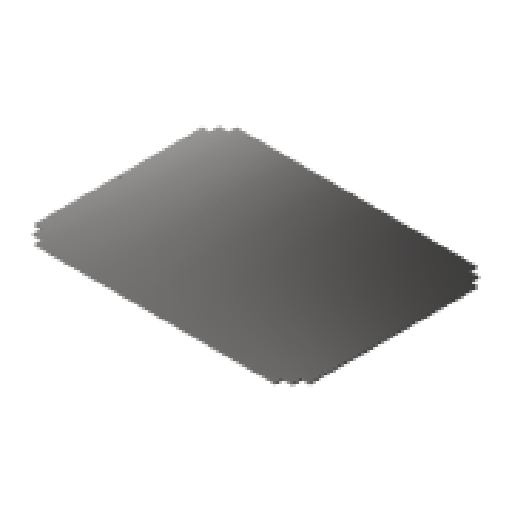
# Autodesk Inventor part: BasePlate
Saved by Autodesk Inventor 2023.2 (Build 272271000, 271)
## iProperties
Created: 2020-05-08
Part Number: BasePlate
Material: Aluminum 6061
Document SubType Name: Modeling
Designer: Remo
Mass: 4435.74 g
Surface Area: 3861.35 cm^2
Volume: 565.063 cm^3
Density: 2.7 g/cm^3
Appearance: Aluminum - Dark
Description: LaserTeileOnline / 3mm Aluminum / Base Plate
Author: Remo
Revision Number: 1
Autodesk Inventor part; units mm, degrees
ref_plane "YZ Plane" through (0, 0, 0) normal (1, 0, 0) x (0, 1, 0)
ref_plane "XZ Plane" through (0, 0, 0) normal (0, 1, 0) x (-1, 0, 0)
ref_plane "XY Plane" through (0, 0, 0) normal (0, 0, 1) x (1, 0, 0)
sketch "Sketch1" plane through (0, 0, 0) normal (0, 0, 1) x (1, 0, 0)
  line L0 (-412.8165, 301.8597) -> (87.1835, 301.8597) projected
  line L1 (-427.8165, 301.8597) -> (-412.8165, 301.8597) projected
  line L2 (-427.8165, 286.8597) -> (-427.8165, 301.8597) projected
  line L3 (-427.8165, -73.1403) -> (-427.8165, 286.8597) projected
  line L4 (-412.8165, 286.8597) -> (-427.8165, 286.8597) projected
  line L5 (-412.8165, 286.8597) -> (-427.8165, 286.8597) projected
  line L6 (-412.8165, 301.8597) -> (-412.8165, 286.8597) projected
  line L7 (-427.8165, 301.8597) -> (-412.8165, 301.8597) projected
  line L8 (-427.8165, 286.8597) -> (-427.8165, 301.8597) projected
  line L9 (-412.8165, -88.1403) -> (-412.8165, -73.1403) projected
  line L10 (-412.8165, -73.1403) -> (-427.8165, -73.1403) projected
  line L11 (-427.8165, -88.1403) -> (-427.8165, -73.1403) projected
  line L12 (-412.8165, -88.1403) -> (-427.8165, -88.1403) projected
  line L13 (-412.8165, -73.1403) -> (-412.8165, 286.8597) projected
  line L14 (87.1835, -73.1403) -> (-412.8165, -73.1403) projected
  line L15 (87.1835, -88.1403) -> (-412.8165, -88.1403) projected
  line L16 (102.1835, -88.1403) -> (102.1835, -73.1403) projected
  line L17 (102.1835, -73.1403) -> (87.1835, -73.1403) projected
  line L18 (87.1835, -88.1403) -> (87.1835, -73.1403) projected
  line L19 (102.1835, -88.1403) -> (87.1835, -88.1403) projected
  line L20 (87.1835, -73.1403) -> (87.1835, 286.8597) projected
  line L21 (102.1835, -73.1403) -> (102.1835, 286.8597) projected
  line L22 (87.1835, 286.8597) -> (102.1835, 286.8597) projected
  line L23 (102.1835, 286.8597) -> (102.1835, 301.8597) projected
  line L24 (87.1835, 301.8597) -> (102.1835, 301.8597) projected
  line L25 (87.1835, 286.8597) -> (87.1835, 301.8597) projected
  line L26 (87.1835, 286.8597) -> (-412.8165, 286.8597) projected
  line L27 (-312.8165, -73.1403) -> (-312.8165, 286.8597) projected
  line L28 (-297.8165, -73.1403) -> (-297.8165, 286.8597) projected
  line L29 (-12.8165, -73.1403) -> (-12.8165, 286.8597) projected
  line L30 (-27.8165, -73.1403) -> (-27.8165, 286.8597) projected
  line L31 (-425.8165, -71.1403) -> (-410.8165, -71.1403)
  line L32 (-410.8165, -71.1403) -> (-410.8165, -86.1403)
  line L33 (-410.8165, -86.1403) -> (85.1835, -86.1403)
  line L34 (85.1835, -86.1403) -> (85.1835, -71.1403)
  line L35 (85.1835, -71.1403) -> (100.1835, -71.1403)
  line L36 (100.1835, -71.1403) -> (100.1835, 284.8597)
  line L37 (100.1835, 284.8597) -> (85.1835, 284.8597)
  line L38 (85.1835, 284.8597) -> (85.1835, 299.8597)
  line L39 (85.1835, 299.8597) -> (-410.8165, 299.8597)
  line L40 (-410.8165, 299.8597) -> (-410.8165, 284.8597)
  line L41 (-410.8165, 284.8597) -> (-425.8165, 284.8597)
  line L42 (-425.8165, 284.8597) -> (-425.8165, -71.1403)
  point P0 (0, 0)
  dimension "d2" = 2
  dimension "d3" = 2
  dimension "d4" = 2
  dimension "d5" = 2
  dimension "d6" = 2
  dimension "d7" = 2
  dimension "d8" = 2
  dimension "d9" = 2
  dimension "d10" = 2
  dimension "d11" = 2
  dimension "d12" = 2
  dimension "d13" = 2
  constraints: 24 end point, 7 perpendicular, 4 parallel, 1 horizontal
  measures "d2" distance between parallel lines of L10 L31
  measures "d3" distance between parallel lines of L3 L42
  measures "d4" distance between parallel lines of L9 L32
  measures "d5" distance between parallel lines of L15 L33
  measures "d6" distance between parallel lines of L34 L18
  measures "d7" distance between parallel lines of L17 L35
  measures "d8" distance between parallel lines of L21 L36
  measures "d9" distance between parallel lines of L22 L37
  measures "d10" distance between parallel lines of L25 L38
  measures "d11" distance between parallel lines of L0 L39
  measures "d12" distance between parallel lines of L6 L40
  measures "d13" distance between parallel lines of L4 L41
extrude "Extrusion1" add sketch "Sketch1" along normal blind 3 contours L41 L40 L26 L27 L14 L32 L31 L13 | L13 L31 L42 L41 | L40 L39 L38 L26 | L37 L36 L35 L20 | L20 L35 L34 L14 L29 L26 L38 L37 | L26 L28 L14 L27 | L29 L14 L30 L26 | L26 L30 L14 L28 | L14 L34 L33 L32
sketch "Sketch3" plane through (0, 0, 3) normal (0, 0, 1) x (1, 0, 0)
  line L0 (100.1835, -71.1403) -> (100.1835, 284.8597) projected
  line L1 (-425.8165, 284.8597) -> (-425.8165, -71.1403) projected
  line L2 (-425.8165, -71.1403) -> (-410.8165, -71.1403) projected
  line L3 (-410.8165, 284.8597) -> (-425.8165, 284.8597) projected
  line L4 (85.1835, -86.1403) -> (85.1835, -71.1403) projected
  line L5 (-410.8165, 299.8597) -> (-410.8165, 284.8597) projected
  line L6 (-410.8165, -86.1403) -> (85.1835, -86.1403) projected
  line L7 (85.1835, 299.8597) -> (-410.8165, 299.8597) projected
  point P0 (0, 0)
  point P1 (94.6835, -21.1403)
  point P2 (94.6835, 106.8597)
  point P3 (94.6835, 234.8597)
  point P4 (-420.3165, 234.8597)
  point P5 (-420.3165, 106.8597)
  point P6 (-420.3165, -21.1403)
  point P7 (35.1835, -80.6403)
  point P8 (-94.8165, -80.6403)
  point P9 (-230.8165, -80.6403)
  point P10 (-360.8165, -80.6403)
  point P11 (-360.8165, 294.3597)
  point P12 (-230.8165, 294.3597)
  point P13 (-94.8165, 294.3597)
  point P14 (35.1835, 294.3597)
  dimension "d18" = 5.5
  dimension "d19" = 5.5
  dimension "d20" = 50
  dimension "d21" = 50
  dimension "d22" = 356
  dimension "d23" = 178
  dimension "d24" = 50
  dimension "d25" = 50
  dimension "d26" = 5.5
  dimension "d27" = 5.5
  dimension "d28" = 180
  dimension "d29" = 180
  constraints: 9 horizontal alignment, 8 vertical alignment
  measures "d18" distance from line of L0 point (94.684, -21.14)
  measures "d19" distance from line of L1 point (-420.316, -21.14)
  measures "d20" distance from line of L2 point (-420.316, -21.14)
  measures "d21" distance from line of L3 point (-420.316, 234.86)
  measures "d22" distance of L1.start L1.end
  measures "d23" distance from line of L2 point (-420.316, 106.86)
  measures "d24" distance from line of L4 point (35.184, -80.64)
  measures "d25" distance from line of L5 point (-360.816, 294.36)
  measures "d26" distance from line of L6 point (35.184, -80.64)
  measures "d27" distance from line of L7 point (35.184, 294.36)
  measures "d28" horizontal distance of L6.start point (-230.816, -80.64)
  measures "d29" distance from line of L4 point (-94.816, -80.64)
hole "FrameMountHoles" at (94.6835, -21.1403, 3) at (94.6835, 106.8597, 3) at (94.6835, 234.8597, 3) at (-420.3165, 234.8597, 3) at (-420.3165, 106.8597, 3) at (-420.3165, -21.1403, 3) at (35.1835, -80.6403, 3) at (-94.8165, -80.6403, 3) at (-230.8165, -80.6403, 3) at (-360.8165, -80.6403, 3) at (-360.8165, 294.3597, 3) at (-230.8165, 294.3597, 3) at (-94.8165, 294.3597, 3) at (35.1835, 294.3597, 3) direction (0, 0, -1) diameter 4 depth 8 tip angle 118
sketch "Sketch10" plane through (0, 0, 3) normal (0, 0, 1) x (1, 0, 0)
  circle A0 centre (-94.8165, 294.3597) radius 2 projected
  circle A1 centre (-360.8165, 294.3597) radius 2 projected
  circle A2 centre (-230.8165, -80.6403) radius 2 projected
  circle A3 centre (35.1835, -80.6403) radius 2 projected
  circle A4 centre (-420.3165, 106.8597) radius 2 projected
  circle A5 centre (94.6835, 234.8597) radius 2 projected
  circle A6 centre (94.6835, -21.1403) radius 2 projected
  circle A7 centre (94.6835, 106.8597) radius 2 projected
  circle A8 centre (-420.3165, 234.8597) radius 2 projected
  circle A9 centre (-420.3165, -21.1403) radius 2 projected
  circle A10 centre (-94.8165, -80.6403) radius 2 projected
  circle A11 centre (-360.8165, -80.6403) radius 2 projected
  circle A12 centre (-230.8165, 294.3597) radius 2 projected
  circle A13 centre (35.1835, 294.3597) radius 2 projected
  line L0 (-425.8165, -71.1403) -> (-410.8165, -71.1403) projected
  line L1 (-410.8165, -71.1403) -> (-410.8165, -86.1403) projected
  line L2 (-410.8165, -86.1403) -> (85.1835, -86.1403) projected
  line L3 (85.1835, -86.1403) -> (85.1835, -71.1403) projected
  line L4 (85.1835, -71.1403) -> (100.1835, -71.1403) projected
  line L5 (100.1835, -71.1403) -> (100.1835, 284.8597) projected
  line L6 (100.1835, 284.8597) -> (85.1835, 284.8597) projected
  line L7 (85.1835, 284.8597) -> (85.1835, 299.8597) projected
  line L8 (85.1835, 299.8597) -> (-410.8165, 299.8597) projected
  line L9 (-410.8165, 299.8597) -> (-410.8165, 284.8597) projected
  line L10 (-410.8165, 284.8597) -> (-425.8165, 284.8597) projected
  line L11 (-425.8165, 284.8597) -> (-425.8165, -71.1403) projected
  line L12 (100.1835, -71.1403) -> (100.1835, 284.8597) projected
  line L13 (85.1835, 284.8597) -> (100.1835, 284.8597)
  line L14 (100.1835, 284.8597) -> (100.1835, 266.8597)
  line L15 (100.1835, 266.8597) -> (85.1835, 266.8597)
  line L16 (85.1835, 266.8597) -> (85.1835, 284.8597)
  line L17 (85.1835, 284.8597) -> (67.1835, 284.8597)
  line L18 (67.1835, 284.8597) -> (67.1835, 299.8597)
  line L19 (67.1835, 299.8597) -> (85.1835, 299.8597)
  line L20 (85.1835, 299.8597) -> (85.1835, 284.8597)
  line L21 (-410.8165, 284.8597) -> (-392.8165, 284.8597)
  line L22 (-392.8165, 284.8597) -> (-392.8165, 299.8597)
  line L23 (-392.8165, 299.8597) -> (-410.8165, 299.8597)
  line L24 (-410.8165, 299.8597) -> (-410.8165, 284.8597)
  line L25 (-410.8165, 284.8597) -> (-425.8165, 284.8597)
  line L26 (-425.8165, 284.8597) -> (-425.8165, 266.8597)
  line L27 (-425.8165, 266.8597) -> (-410.8165, 266.8597)
  line L28 (-410.8165, 266.8597) -> (-410.8165, 284.8597)
  line L29 (-410.8165, -71.1403) -> (-425.8165, -71.1403)
  line L30 (-425.8165, -71.1403) -> (-425.8165, -53.1403)
  line L31 (-425.8165, -53.1403) -> (-410.8165, -53.1403)
  line L32 (-410.8165, -53.1403) -> (-410.8165, -71.1403)
  line L33 (-410.8165, -71.1403) -> (-392.8165, -71.1403)
  line L34 (-392.8165, -71.1403) -> (-392.8165, -86.1403)
  line L35 (-392.8165, -86.1403) -> (-410.8165, -86.1403)
  line L36 (-410.8165, -86.1403) -> (-410.8165, -71.1403)
  line L37 (-410.8165, -86.1403) -> (85.1835, -86.1403) projected
  line L38 (85.1835, -71.1403) -> (67.1835, -71.1403)
  line L39 (67.1835, -71.1403) -> (67.1835, -86.1403)
  line L40 (67.1835, -86.1403) -> (85.1835, -86.1403)
  line L41 (85.1835, -86.1403) -> (85.1835, -71.1403)
  line L42 (85.1835, -71.1403) -> (100.1835, -71.1403)
  line L43 (100.1835, -71.1403) -> (100.1835, -53.1403)
  line L44 (100.1835, -53.1403) -> (85.1835, -53.1403)
  line L45 (85.1835, -53.1403) -> (85.1835, -71.1403)
  point P0 (0, 0)
  dimension "d78" = 18
  constraints: 64 end point, 16 parallel, 8 horizontal, 8 perpendicular, 8 point on line, 7 equal length
  measures "d78" distance of L3.end L38.end
extrude "TriCuts" cut sketch "Sketch10" against normal through all contours L11 L31 L32 L0 | L33 L34 L2 L1 | L11 L10 L28 L27 | L39 L38 L3 L2 | L9 L8 L22 L21 | L45 L44 L5 L4 | L8 L7 L17 L18 | L15 L16 L6 L5
equation "\"d4\" = d2"
equation "\"d5\" = d3"
equation "\"d6\" = d2"
equation "\"d7\" = d2"
equation "\"d8\" = d3"
equation "\"d9\" = d2"
equation "\"d10\" = d2"
equation "\"d11\" = d3"
equation "\"d12\" = d2"
equation "\"d13\" = d2"
equation "\"d19\" = d18"
equation "\"d23\" = 0.5 * d22"
equation "\"d26\" = d18"
equation "\"d27\" = d18"
equation "\"d29\" = d28"
body "Solid1"
